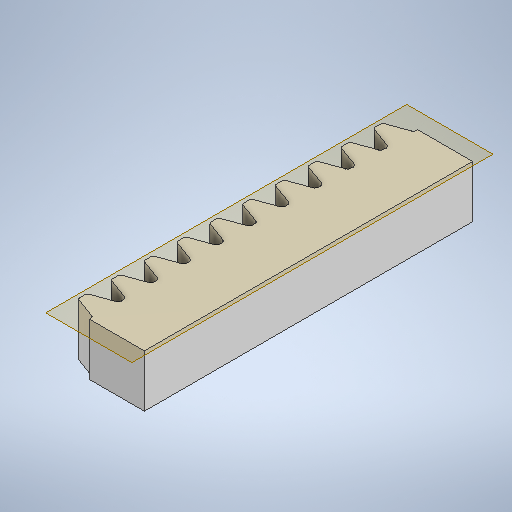
# Autodesk Inventor part: lack1
Saved by Autodesk Inventor 2025.2 (Build 292293000, 293)
## iProperties
Created: 2025-01-11
Part Number: lack1
Material: 一般
Document SubType Name: Modeling
Designer: mahhy
Density: 1 g/cm^3
Appearance: 既定
Author: mahhy
Autodesk Inventor part; units mm, degrees
ref_plane "YZ Plane" through (0, 0, 0) normal (1, 0, 0) x (0, 1, 0)
ref_plane "XZ Plane" through (0, 0, 0) normal (0, 1, 0) x (-1, 0, 0)
ref_plane "XY Plane" through (0, 0, 0) normal (0, 0, 1) x (1, 0, 0)
sketch "スケッチ1" plane through (0, 0, 0) normal (0, 1, 0) x (-1, 0, 0)
  point P0 (0, 0)
  point P1 (4.6985, 0)
  point P2 (6.4922, 1.415)
  constraints: 3 other
sketch "スケッチ2" plane through (0, 0, 0) normal (0, 1, 0) x (-1, 0, 0)
  line L0 (3.75, 15.708) -> (-3.75, 15.708)
  line L1 (-3.75, 15.708) -> (-3.75, -15.708)
  line L2 (-3.75, -15.708) -> (3.75, -15.708)
  line L3 (3.75, -15.708) -> (3.75, 15.708)
  line L4 (3.75, 15.708) -> (-3.75, -15.708)
  line L5 (3.75, -15.708) -> (-3.75, 15.708)
  point P0 (0, 0)
  point P1 (0.0816, -5.789)
  point P2 (0, 0)
  dimension "d2" = 7.5
  dimension "d3" = 31.4159
  constraints: 12 end point, 2 parallel, 1 coincident, 1 horizontal, 1 midpoint, 1 perpendicular
  measures "d2" distance of L2.end L1.end
  measures "d3" distance of L1.end L0.end
extrude "押し出し1" add sketch "スケッチ2" along normal blind 5
ref_plane "作業平面1" through (0, 5, 0) normal (0, 1, 0) x (1, 0, 0)
sketch "スケッチ3" plane through (0, 5, 0) normal (0, 1, 0) x (1, 0, 0)
  line L0 (-3.75, 15.708) -> (-3.75, -15.708) projected
  line L1 (-3.75, -12.5664) -> (3.75, -12.5664)
  line L2 (3.75, -15.708) -> (3.75, 15.708) projected
  line L3 (-3.75, -15.708) -> (3.75, -15.708) projected
  line L4 (-3.75, -14.1372) -> (3.75, -14.1372)
  line L5 (-2.75, -15.708) -> (-2.75, -12.5664)
  line L6 (-1.5, -15.708) -> (-1.5, -12.5664)
  line L7 (-3.75, -14.5586) -> (-1.5, -15.3775)
  line L8 (-3.75, -14.5586) -> (-1.3556, -14.5586) construction
  line L9 (-3.75, -13.7157) -> (-1.5, -12.8968)
  line L10 (-3.75, -13.7157) -> (-1.3556, -13.7157) construction
  point P0 (0, 0)
  point P1 (-2.75, -14.9226)
  point P2 (-2.75, -13.3518)
  dimension "d8" = 1.5708
  dimension "d9" = 1.5708
  dimension "d10" = 1
  dimension "d11" = 1.25
  dimension "d12" = 0.7854
  dimension "d13" = 0.7854
  dimension "d14" = 20
  dimension "d15" = 20
  constraints: 16 end point, 16 point on line, 3 horizontal, 3 perpendicular, 2 equal length
  measures "d8" distance between parallel lines of L4 L3
  measures "d9" distance between parallel lines of L1 L4
  measures "d10" distance between parallel lines of L0 L5
  measures "d11" distance between parallel lines of L5 L6
  measures "d12" distance of L5.start point (-2.75, -14.923)
  measures "d13" distance from line of L4 point (-2.75, -13.352)
  measures "d14" angle of L7 L8
  measures "d15" angle of L10 L9
extrude "押し出し2" cut sketch "スケッチ3" against normal blind 5 contours L1 L5 L9 L0 | L1 L6 L9 L5 | L7 L5 L3 L0 | L7 L6 L3 L5
fillet "フィレット1" radius 0.3 2 edges at (-1.5, 2.5, 12.8968) (-1.5, 2.5, 15.3775)
chamfer "面取り1" distance 0.1 angle 45 2 edges at (-3.75, 2.5, 14.5586) (-3.75, 2.5, 13.7157)
pattern_linear "矩形状パターン1" count 10 spacing 3.1416 along (0, 0, -1) of "押し出し2", "面取り1", "フィレット1"
equation "\"module\" = 1"
